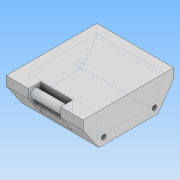
# Autodesk Inventor part: 車身
Saved by Autodesk Inventor 2021 (Build 250183000, 183)
## iProperties
Created: 2025-12-12
Part Number: 車身
Material: 一般
Document SubType Name: Modeling
Designer: User
Density: 1 g/cm^3
Appearance: 預設
Author: User
Autodesk Inventor part; units mm, degrees
ref_plane "YZ Plane" through (0, 0, 0) normal (1, 0, 0) x (0, 1, 0)
ref_plane "XZ Plane" through (0, 0, 0) normal (0, 1, 0) x (-1, 0, 0)
sketch "草圖1" plane through (0, 0, 0) normal (1, 0, 0) x (0, 1, 0)
  line L0 (500, 1000) -> (500, -1000)
  line L1 (0, 650) -> (0, -650)
  line L2 (0, -650) -> (500, -1000)
  line L3 (0, 650) -> (500, 1000)
  line L4 (500, 1000) -> (700, 1000)
  line L5 (700, 1000) -> (700, -1000)
  line L6 (700, -1000) -> (500, -1000)
  line L7 (500, -1000) -> (500, 1000)
  circle A0 centre (560, 875) radius 90
  line L8 (785.0874, 735) -> (28.1159, 735)
  point P0 (0, 0)
  point P1 (0, 0)
  point P2 (500, 0)
  point P3 (700, 735)
  point P4 (560, 785)
  point P5 (121.4286, 735)
  point P6 (500, 735)
  point P7 (500, 807.918)
  point P8 (500, 942.082)
  dimension "d0" = 1300
  dimension "d1" = 2000
  dimension "d2" = 500
  dimension "d3" = 200
  dimension "d6" = 180
  dimension "d7" = 140
  dimension "d8" = 125
  dimension "d32" = 265
  constraints: 19 end point, 2 horizontal, 2 midpoint, 2 parallel, 2 vertical, 1 centre point, 1 coincident, 1 horizontal alignment, 1 perpendicular
  measures "d0" distance of L1.start L1.end
  measures "d1" distance of L0.start L0.end
  measures "d2" horizontal distance of L1.end L0.end
  measures "d3" distance of L5.end L0.end
  measures "d6" diameter of A0
  measures "d7" distance from line of L5 A0.centre
  measures "d8" distance from line of L4 A0.centre
  measures "d32" distance between parallel lines of L8 L4
extrude "擠出1" add sketch "草圖1" along normal mid plane 1700 contours A0 L0 | L0 A0 | L8 L0 L2 L1 L3 | L8 L5 L6 L0
extrude "擠出2" add sketch "草圖1" against normal blind 500 from surface at 850 contours L4 L5 L8 L0 A0 | L0 A0 L8 L3 | A0 L0 | L0 A0 | L8 L0 L2 L1 L3
extrude "擠出3" add sketch "草圖1" along normal blind 500 from surface at -850 contours L4 L5 L8 L0 A0 | L0 A0 L8 L3 | A0 L0 | L0 A0 | L8 L0 L2 L1 L3
sketch "草圖2" plane through (-350, 560, 875) normal (1, 0, 0) x (0, 0, -1)
  circle A0 centre (10, -180) radius 22.5
  line L0 (140, -438.5714) -> (140, 140) projected
  line L1 (-125, 140) -> (140, 140) projected
  line L2 (-125, -60) -> (-125, 140) projected
  line L3 (140, -438.5714) -> (-125, -60) projected
  line L4 (225, -560) -> (140, -438.5714) projected
  line L5 (1525, -560) -> (225, -560) projected
  line L6 (1875, -60) -> (1525, -560) projected
  line L7 (1875, 140) -> (1875, -60) projected
  line L8 (140, 140) -> (1875, 140) projected
  circle A1 centre (0, 0) radius 90 projected
  point P0 (875, -560)
  dimension "d13" = 45
  dimension "d15" = 320
  constraints: 1 centre point
  measures "d13" diameter of A0
  measures "d15" distance from line of L1 A0.centre
extrude "擠出4" add sketch "草圖2" along normal up to next contours A0
ref_plane "工作平面1" through (750, 0, 0) normal (1, 0, 0) x (0, 0, -1)
sketch "草圖4" plane through (750, 0, 0) normal (1, 0, 0) x (0, 0, -1)
  line L0 (-1000, 700) -> (1000, 700) projected
  line L1 (1000, 700) -> (1000, 500) projected
  line L2 (1000, 500) -> (650, 0) projected
  line L3 (650, 0) -> (-650, 0) projected
  line L4 (-650, 0) -> (-1000, 500) projected
  line L5 (-1000, 500) -> (-1000, 700) projected
  line L6 (597.9344, 100) -> (900, 531.5222)
  line L7 (900, 531.5222) -> (900, 600)
  line L8 (900, 600) -> (-900, 600)
  line L9 (-900, 600) -> (-900, 531.5222)
  line L10 (-900, 531.5222) -> (-597.9344, 100)
  line L11 (-597.9344, 100) -> (597.9344, 100)
  line L12 (-597.9344, 1100.1132) -> (-597.9344, -380.0313)
  point P0 (0, 0)
  point P1 (-597.9344, 600)
  dimension "d20" = 100
  constraints: 14 end point, 1 point on line, 1 vertical, 5 other
  measures "d20" distance between parallel lines of L2 L6
extrude "擠出5" cut sketch "草圖4" against normal blind 1500 contours L8 L7 L6 L11 L12
sketch "草圖5" plane through (850, 0, 0) normal (1, 0, 0) x (0, 0, -1)
  circle A0 centre (-547.9344, 150) radius 50
  circle A1 centre (571.9017, 150) radius 50
  line L0 (-650, 0) -> (650, 0) projected
  line L1 (-597.9344, 600) -> (-597.9344, 100) projected
  line L2 (-597.9344, 100) -> (597.9344, 100) projected
  line L3 (597.9344, 100) -> (900, 531.5222) projected
  point P0 (0, 0)
  dimension "d24" = 100
  dimension "d25" = 100
  constraints: 4 tangent, 2 centre point
  measures "d24" diameter of A0
  measures "d25" diameter of A1
extrude "擠出6" cut sketch "草圖5" against normal through all contours A0 | A1
thread "螺紋2" size "1 13/16-6 UN" class "2A" standard "ANSI Unified Screw Threads" full length
equation "\"d25\" = d24"
